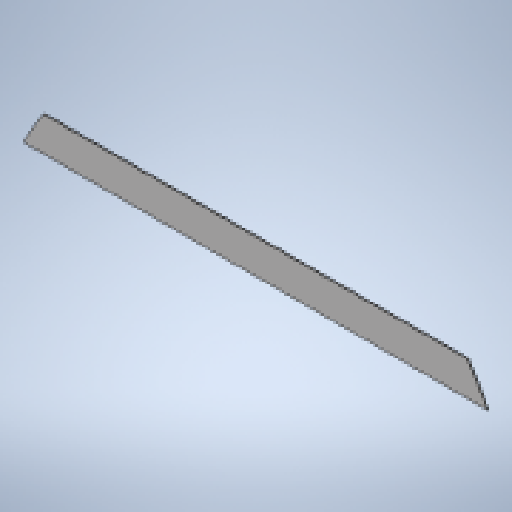
# Autodesk Inventor part: MSC 201 GRID
Saved by Autodesk Inventor 2025 (Build 290162010, 162A)
## iProperties
Created: 2025-01-14
Part Number: MSC 201 GRID
Material: Stainless Steel
Document SubType Name: Sheet Metal
Designer: pokla
Density: 8 g/cm^3
Sheet Metal Rule: AISI304 3mm Die 32
Appearance: Default
Author: pokla
Autodesk Inventor part; units mm, degrees
ref_plane "YZ Plane" through (0, 0, 0) normal (1, 0, 0) x (0, 1, 0)
ref_plane "XZ Plane" through (0, 0, 0) normal (0, 1, 0) x (-1, 0, 0)
ref_plane "XY Plane" through (0, 0, 0) normal (0, 0, 1) x (1, 0, 0)
sketch "Sketch1" plane through (0, 0, 0) normal (0, 1, 0) x (-1, 0, 0)
  line L0 (900, 50) -> (-900, 50)
  line L1 (-900, 50) -> (-900, -50)
  line L2 (-900, -50) -> (900, -50)
  line L3 (900, -50) -> (900, 50)
  line L4 (900, 50) -> (-900, -50) construction
  line L5 (676.9, 50) -> (734.5885, -50)
  line L6 (0, 50) -> (0, -50) construction
  line L7 (-676.9, 50) -> (-734.5885, -50)
  point P0 (0, 0)
  point P1 (0, 0)
  dimension "d0" = 100
  dimension "d1" = 1800
  dimension "d3" = 119.98
  dimension "d6" = 676.9
  dimension "d7" = 119.98
  dimension "d8" = 676.9
  measures "d0" distance of L2.end L0.start
  measures "d1" distance of L0.start L0.end
  measures "d3" angle of L0 L5
  measures "d6" distance of L6.start L5.start
  measures "d7" angle of L0 L7
  measures "d8" distance of L6.start L7.start
extrude "Plate1" add sketch "Sketch1" along normal mid plane 3 contours L5 L2 L7 L0
equation "\"d7\" = d3"
equation "\"d8\" = d6"
equation "\"d2\" = Thickness"
equation "\"BendReliefWidth\" = Thickness"
equation "\"BendReliefDepth\" = 0.5 * Thickness"
equation "\"CornerReliefSize\" = 4 * Thickness"
equation "\"MinimumRemnant\" = 2 * Thickness"
equation "\"TransitionRadius\" = BendRadius"
equation "\"JacobiRadiusSize\" = BendRadius"
equation "\"GapSize\" = Thickness"
equation "\"Thickness\" = 3"
equation "\"BendRadius\" = 5"
body "Solid1"
